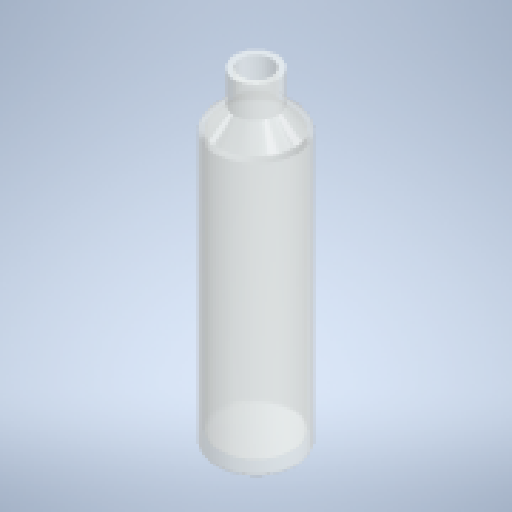
# Autodesk Inventor part: Bouteille
Saved by Autodesk Inventor 2024.2 (Build 282272000, 272)
## iProperties
Created: 2024-09-10
Part Number: Bouteille
Material: Verre
Document SubType Name: Modeling
Designer: Sebastien
Density: 2.18 g/cm^3
Appearance: Clair
Author: Sebastien
Autodesk Inventor part; units mm, degrees
ref_plane "YZ Plane" through (0, 0, 0) normal (1, 0, 0) x (0, 1, 0)
ref_plane "XZ Plane" through (0, 0, 0) normal (0, 1, 0) x (-1, 0, 0)
ref_plane "XY Plane" through (0, 0, 0) normal (0, 0, 1) x (1, 0, 0)
sketch "Esquisse1" plane through (0, 0, 0) normal (0, 0, 1) x (1, 0, 0)
  line L0 (0, 8) -> (0, 5)
  arc A0 (24.3671, 0.2221) -> (0, 5) centre (0, -59.525) ccw
  arc A1 (24.3671, 0.2221) -> (28.5, 3) centre (25.5, 3) ccw
  line L1 (28.5, 3) -> (28.5, 189.1581)
  arc A2 (28.5, 189.1581) -> (27.143, 192.5828) centre (23.5, 189.1581) ccw
  line L2 (27.143, 192.5828) -> (15, 205.5)
  line L3 (15, 205.5) -> (15, 227)
  line L4 (15, 227) -> (10.75, 227)
  line L5 (10.75, 227) -> (10.75, 207.6222)
  arc A3 (10.75, 207.6222) -> (12.107, 204.1975) centre (15.75, 207.6222) ccw
  line L6 (12.107, 204.1975) -> (24.143, 191.3941)
  arc A4 (25.5, 187.9694) -> (24.143, 191.3941) centre (20.5, 187.9694) ccw
  line L7 (25.5, 187.9694) -> (25.5, 10)
  arc A5 (23.5, 8) -> (25.5, 10) centre (23.5, 10) ccw
  line L8 (23.5, 8) -> (0, 8)
  line L9 (0, 0) -> (25.5, 0) construction
  point P0 (28.1484, 191)
  dimension "d0" = 57
  dimension "d1" = 30
  dimension "d2" = 21.5
  dimension "d3" = 21.5
  dimension "d4" = 3
  dimension "d5" = 3
  dimension "d6" = 14.5
  dimension "d7" = 5
  dimension "d8" = 3
  dimension "d9" = 3
  dimension "d10" = 2
  dimension "d11" = 227
  dimension "d12" = 5
  constraints: 21 end point, 14 point on circle, 11 tangent, 6 centre point, 3 parallel, 2 equal radius, 2 horizontal, 2 perpendicular, 2 vertical, 1 point on line, 1 vertical alignment
  measures "d0" diameter of L1 L0
  measures "d1" diameter of L3 L0
  measures "d2" diameter of L5 L0
  measures "d3" distance from line of L2.end L4
  measures "d4" distance between parallel lines of L6 L2
  measures "d5" distance between parallel lines of L1 L7
  measures "d6" vertical distance of point (28.148, 191) L2.end
  measures "d7" distance from line of L9 L0.end
  measures "d8" radius of A1
  measures "d9" distance of L0.start L0.end
  measures "d10" radius of A5
  measures "d11" distance between parallel lines of L9 L4
  measures "d12" radius of A2
revolve "Révolution1" add sketch "Esquisse1" angle 360 about axis through (0, 8, 0) along (0, -1, 0)
equation "\"d5\" = d4"
